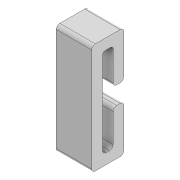
# Autodesk Inventor part: ruziiiii
Saved by Autodesk Inventor 2020 (Build 240168000, 168)
## iProperties
Created: 2025-05-22
Part Number: ruziiiii
Material: Типовые
Document SubType Name: Modeling
Designer: 4s
Density: 1 g/cm^3
Appearance: По умолчанию
Author: 4s
## iProperties of the stored document _3DПЕЧАТЬ.ipt
Created: 2025-05-22
Part Number: _3DПЕЧАТЬ
Material: Типовые
Document SubType Name: Modeling
Designer: 4s
Density: 1 g/cm^3
Appearance: По умолчанию
Author: 4s
Autodesk Inventor part; units mm, degrees
ref_plane "YZ Plane" through (0, 0, 0) normal (1, 0, 0) x (0, 1, 0)
ref_plane "XZ Plane" through (0, 0, 0) normal (0, 1, 0) x (-1, 0, 0)
ref_plane "XY Plane" through (0, 0, 0) normal (0, 0, 1) x (1, 0, 0)
sketch "Эскиз1" plane through (0, 0, 0) normal (1, 0, 0) x (0, 1, 0)
  line L0 (-0.75, 0) -> (-24, 0)
  line L1 (-25, -1) -> (-25, -2)
  line L2 (0, -2.25) -> (0, -0.75)
  line L3 (2, 3) -> (-27, 3)
  line L4 (-28, 2) -> (-28, -5)
  line L5 (3, -5) -> (3, 2)
  line L6 (-15, -4) -> (-15, -5)
  line L7 (-10, -5) -> (-10, -4)
  arc A0 (2, -6) -> (3, -5) centre (2, -5) ccw
  arc A1 (3, 2) -> (2, 3) centre (2, 2) ccw
  arc A2 (-27, 3) -> (-28, 2) centre (-27, 2) ccw
  arc A3 (-28, -5) -> (-27, -6) centre (-27, -5) ccw
  arc A4 (-25, -2) -> (-24, -3) centre (-24, -2) ccw
  arc A5 (-24, 0) -> (-25, -1) centre (-24, -1) ccw
  arc A6 (0, -0.75) -> (-0.75, 0) centre (-0.75, -0.75) ccw
  arc A7 (-0.75, -3) -> (0, -2.25) centre (-0.75, -2.25) ccw
  line L8 (-0.4776, -6) -> (-9, -6)
  line L9 (-16, -6) -> (-17.3462, -6)
  line L10 (-24, -3) -> (-16, -3)
  line L11 (-9, -3) -> (-0.75, -3)
  line L12 (-27, -6) -> (-16, -6)
  line L13 (-9, -6) -> (2, -6)
  arc A8 (-9, -3) -> (-10, -4) centre (-9, -4) ccw
  arc A9 (-10, -5) -> (-9, -6) centre (-9, -5) ccw
  arc A10 (-15, -4) -> (-16, -3) centre (-16, -4) ccw
  arc A11 (-16, -6) -> (-15, -5) centre (-16, -5) ccw
  line L14 (2, -5) -> (-27, 2) construction
  line L15 (2, 2) -> (-27, -5) construction
  line L16 (-10, -4) -> (3, -4) construction
  line L17 (-15, -4) -> (-28, -4) construction
  point P0 (0, 0)
  point P1 (-25, -3)
  point P2 (-25, 0)
  point P3 (0, -3)
  dimension "d1" = 3
  dimension "d4" = 3
  dimension "d5" = 3
  dimension "d6" = 3
  dimension "d7" = 5
  dimension "d8" = 1
  dimension "d9" = 0.75
  dimension "d10" = 13
  dimension "d11" = 1
  dimension "d12" = 1
  dimension "d15" = 3
  dimension "d16" = 25
  constraints: 36 end point, 28 tangent, 24 point on circle, 12 centre point, 11 parallel, 8 equal radius, 8 point on line, 4 perpendicular, 2 horizontal, 1 collinear
  measures "d1" distance of point (-25, -3) point (-25, 0)
  measures "d4" distance between parallel lines of L0 L3
  measures "d5" distance between parallel lines of L5 L2
  measures "d6" distance between parallel lines of L1 L4
  measures "d7" distance between parallel lines of L6 L7
  measures "d8" radius of A0
  measures "d9" radius of A6
  measures "d10" distance between parallel lines of L5 L7
  measures "d11" radius of A8
  measures "d12" radius of A10
  measures "d15" distance between parallel lines of L13 L11
  measures "d16" distance between parallel lines of L1 L2
extrude "Выдавливание1" add sketch "Эскиз1" along normal blind 10
